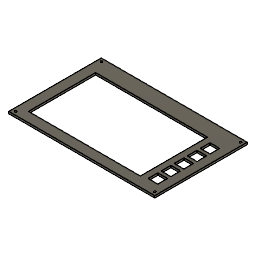
Case_plate_source (Autodesk Fusion 360 archive; units mm, degrees)
design "Case_top"
Autodesk Fusion 360 part; units mm, degrees
sketch "plate-2026-03-03T15_18_35.082Z" plane through (0, 0, 0) normal (0, 0, 1) x (1, 0, 0)
  line L0 (-7.0864, -44.9336) -> (-7.0864, -31.9336)
  line L1 (6.9136, -44.9336) -> (6.9136, -31.9336)
  line L2 (-6.5864, -45.4336) -> (6.4136, -45.4336)
  line L3 (-6.5864, -31.4336) -> (6.4136, -31.4336)
  arc A0 (-7.0864, -44.9336) -> (-6.5864, -45.4336) centre (-6.5864, -44.9336) ccw
  arc A1 (-6.5864, -31.4336) -> (-7.0864, -31.9336) centre (-6.5864, -31.9336) ccw
  arc A2 (6.4136, -45.4336) -> (6.9136, -44.9336) centre (6.4136, -44.9336) ccw
  arc A3 (6.9136, -31.9336) -> (6.4136, -31.4336) centre (6.4136, -31.9336) ccw
  line L4 (-7.0864, -25.8836) -> (-7.0864, -12.8836)
  line L5 (6.9136, -25.8836) -> (6.9136, -12.8836)
  line L6 (-6.5864, -26.3836) -> (6.4136, -26.3836)
  line L7 (-6.5864, -12.3836) -> (6.4136, -12.3836)
  arc A4 (-7.0864, -25.8836) -> (-6.5864, -26.3836) centre (-6.5864, -25.8836) ccw
  arc A5 (-6.5864, -12.3836) -> (-7.0864, -12.8836) centre (-6.5864, -12.8836) ccw
  arc A6 (6.4136, -26.3836) -> (6.9136, -25.8836) centre (6.4136, -25.8836) ccw
  arc A7 (6.9136, -12.8836) -> (6.4136, -12.3836) centre (6.4136, -12.8836) ccw
  line L8 (-7.0864, -6.8336) -> (-7.0864, 6.1664)
  line L9 (6.9136, -6.8336) -> (6.9136, 6.1664)
  line L10 (-6.5864, -7.3336) -> (6.4136, -7.3336)
  line L11 (-6.5864, 6.6664) -> (6.4136, 6.6664)
  arc A8 (-7.0864, -6.8336) -> (-6.5864, -7.3336) centre (-6.5864, -6.8336) ccw
  arc A9 (-6.5864, 6.6664) -> (-7.0864, 6.1664) centre (-6.5864, 6.1664) ccw
  arc A10 (6.4136, -7.3336) -> (6.9136, -6.8336) centre (6.4136, -6.8336) ccw
  arc A11 (6.9136, 6.1664) -> (6.4136, 6.6664) centre (6.4136, 6.1664) ccw
  line L12 (-7.0864, 12.2164) -> (-7.0864, 25.2164)
  line L13 (6.9136, 12.2164) -> (6.9136, 25.2164)
  line L14 (-6.5864, 11.7164) -> (6.4136, 11.7164)
  line L15 (-6.5864, 25.7164) -> (6.4136, 25.7164)
  arc A12 (-7.0864, 12.2164) -> (-6.5864, 11.7164) centre (-6.5864, 12.2164) ccw
  arc A13 (-6.5864, 25.7164) -> (-7.0864, 25.2164) centre (-6.5864, 25.2164) ccw
  arc A14 (6.4136, 11.7164) -> (6.9136, 12.2164) centre (6.4136, 12.2164) ccw
  arc A15 (6.9136, 25.2164) -> (6.4136, 25.7164) centre (6.4136, 25.2164) ccw
  line L16 (-7.0864, 31.2664) -> (-7.0864, 44.2664)
  line L17 (6.9136, 31.2664) -> (6.9136, 44.2664)
  line L18 (-6.5864, 30.7664) -> (6.4136, 30.7664)
  line L19 (-6.5864, 44.7664) -> (6.4136, 44.7664)
  arc A16 (-7.0864, 31.2664) -> (-6.5864, 30.7664) centre (-6.5864, 31.2664) ccw
  arc A17 (-6.5864, 44.7664) -> (-7.0864, 44.2664) centre (-6.5864, 44.2664) ccw
  arc A18 (6.4136, 30.7664) -> (6.9136, 31.2664) centre (6.4136, 31.2664) ccw
  arc A19 (6.9136, 44.2664) -> (6.4136, 44.7664) centre (6.4136, 44.2664) ccw
  line L20 (9.4386, -47.9586) -> (9.4386, 47.2914)
  line L21 (-9.6114, -47.9586) -> (-9.6114, 47.2914)
  line L22 (9.4386, -47.9586) -> (-9.6114, -47.9586)
  line L23 (9.4386, 47.2914) -> (-9.6114, 47.2914)
sketch "Sketch2" plane through (0, 0, 0) normal (0, 0, 1) x (1, 0, 0)
  line L0 (19.4386, 72.7414) -> (-193.7614, 72.7414)
  line L1 (-193.7614, 72.7414) -> (-193.7614, -62.4586)
  line L2 (-193.7614, -62.4586) -> (19.4386, -62.4586)
  line L3 (19.4386, -62.4586) -> (19.4386, 72.7414)
  line L4 (9.4386, -47.9586) -> (9.4386, 47.2914)
  line L5 (9.4386, -47.9586) -> (-9.6114, -47.9586)
  circle A0 centre (14.4386, 67.7414) radius 1.45
  circle A1 centre (-188.7614, 67.7414) radius 1.45
  circle A2 centre (-188.7614, -57.4586) radius 1.45
  circle A3 centre (14.4386, -57.4586) radius 1.45
  line L6 (-179.2614, 49.9614) -> (-16.0614, 49.9614)
  line L7 (-16.0614, 49.9614) -> (-16.0614, -47.9586)
  line L8 (-16.0614, -47.9586) -> (-179.2614, -47.9586)
  line L9 (-179.2614, -47.9586) -> (-179.2614, 49.9614)
  dimension "d1" = 213.2
  dimension "d2" = 135.2
  dimension "d3" = 10
  dimension "d5" = 2.9
  dimension "d6" = 2.9
  dimension "d7" = 2.9
  dimension "d8" = 2.9
  dimension "d9" = 5
  dimension "d10" = 5
  dimension "d11" = 5
  dimension "d12" = 5
  dimension "d13" = 5
  dimension "d14" = 5
  dimension "d15" = 5
  dimension "d16" = 5
  dimension "d17" = 163.2
  dimension "d18" = 97.92
  dimension "d20" = 14.5
  dimension "d22" = 14.5
  dimension "d23" = 14.5
  constraint horizontal L0
  constraint vertical L1
  constraint horizontal L2
  constraint vertical L3
  constraint horizontal L6
  constraint vertical L7
  constraint horizontal L8
  constraint vertical L9
  measures "d1" distance of L0.start L0.end
  measures "d2" distance of L0.start L2.end
  measures "d3" distance of L3 L4
  measures "d5" diameter of A0
  measures "d6" diameter of A1
  measures "d7" diameter of A2
  measures "d8" diameter of A3
  measures "d9" distance of L2 A3.centre
  measures "d10" distance of L3 A3.centre
  measures "d11" distance of L0 A0.centre
  measures "d12" distance of L3 A0.centre
  measures "d13" distance of L0 A1.centre
  measures "d14" distance of L1 A1.centre
  measures "d15" distance of L2 A2.centre
  measures "d16" distance of L1 A2.centre
  measures "d17" distance of L6.start L6.end
  measures "d18" distance of L6.start L8.end
  measures "d20" distance of L1 L9
  measures "d22" distance of L2 L8
  measures "d23" distance of L2 L5
extrude "Extrude1" add sketch "Sketch2" along normal blind 3
extrude "Extrude2" cut sketch "plate-2026-03-03T15_18_35.082Z" along normal blind 15 contours L0 L1 L2 L3 A0 A1 A2 A3 | L4 L5 L6 L7 A4 A5 A6 A7 | L8 L9 L10 L11 A8 A9 A10 A11 | L12 L13 L14 L15 A12 A13 A14 A15 | L16 L17 L18 L19 A16 A17 A18 A19
equation "d1 = 193.2 mm + 20 mm"
equation "d2 = 115.2 mm + 20 mm"
